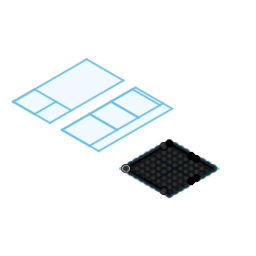
micromouse maze one quarter cutout (Autodesk Fusion 360 design; units mm, degrees)
Autodesk Fusion 360 part; units mm, degrees
sketch "Sketch1" plane through (0, 0, 0) normal (0, 0, 1) x (1, 0, 0)
  line L0 (0, 0) -> (1440, 0)
  line L1 (1440, 0) -> (1440, 1440)
  line L2 (1440, 1440) -> (0, 1440)
  line L3 (0, 1440) -> (0, 0)
  line L4 (720, 1620) -> (720, -180)
  line L5 (0, 0) -> (180, 0)
  line L6 (180, 0) -> (180, 180)
  line L7 (180, 180) -> (0, 180)
  line L8 (0, 180) -> (0, 0)
  line L9 (0, 0) -> (0, -100)
  line L10 (0, -100) -> (-100, -100)
  line L11 (1440, 1440) -> (1540, 1440)
  line L12 (1540, 1440) -> (1540, 1540)
  dimension "d1" = 1440
  dimension "d2" = 1440
  dimension "d7" = 180
  dimension "d8" = 180
  dimension "d9" = 100
  dimension "d10" = 100
  dimension "d11" = 100
  dimension "d12" = 100
  constraint horizontal L0
  constraint vertical L1
  constraint horizontal L2
  constraint vertical L3
  constraint coincident L0.start L3.end
  constraint horizontal L5
  constraint vertical L6
  constraint horizontal L7
  constraint vertical L8
  constraint perpendicular L5 L9
  constraint perpendicular L9 L10
  constraint perpendicular L1 L11
  constraint perpendicular L11 L12
  measures "d1" distance of L0.start L0.end
  measures "d2" distance of L0.start L2.end
  measures "d7" distance of L0.start L5.end
  measures "d8" distance of L0.start L7.end
  measures "d9" distance of L0.start L9.end
  measures "d10" distance of L9.end L10.end
  measures "d11" distance of L1.end L11.end
  measures "d12" distance of L11.end L12.end
extrude "Extrude1" add sketch "Sketch1" along normal blind 12.7
sketch "Sketch2" plane through (0, 0, 12.7) normal (0, 0, 1) x (-1, 0, 0)
  line L0 (0, -1440) -> (0, 0)
  line L1 (0, 0) -> (-1440, 0)
  line L2 (-1440, 0) -> (-1440, -1440)
  line L3 (-1440, -1440) -> (0, -1440)
  line L4 (0, 0) -> (-180, 0)
  line L5 (-180, 0) -> (-360, 0)
  line L6 (-360, 0) -> (-540, 0)
  line L7 (-540, 0) -> (-720, 0)
  line L8 (-720, 0) -> (-720, -1440)
  line L9 (-180, 0) -> (-180, -1440)
  line L10 (-360, 0) -> (-360, -1440)
  line L11 (-540, 0) -> (-540, -1440)
  dimension "d15" = 180
  dimension "d16" = 180
  dimension "d17" = 180
  dimension "d18" = 180
  constraint coincident L0.end L1.start
  constraint perpendicular L0 L4
  constraint perpendicular L0 L5
  constraint parallel L1 L6
  constraint parallel L1 L7
  constraint midpoint L3 L8.end
  constraint coincident L3 L9.end
  constraint perpendicular L3 L9
  constraint coincident L3 L10.end
  constraint perpendicular L3 L10
  constraint coincident L3 L11.end
  constraint perpendicular L3 L11
  measures "d15" distance of L0.end L4.end
  measures "d16" distance of L4.end L5.end
  measures "d17" distance of L5.end L6.end
  measures "d18" distance of L6.end L7.end
sketch "Sketch3" plane through (0, 0, 12.7) normal (0, 0, 1) x (-1, 0, 0)
sketch "Sketch4" plane through (0, 0, 12.7) normal (0, 0, 1) x (-1, 0, 0)
  line L0 (0, 0) -> (-1440, 0)
  line L1 (-1440, 0) -> (-1440, -1440)
  line L2 (-1440, -1440) -> (0, -1440)
  line L3 (0, -1440) -> (0, 0)
  line L4 (-720, 0) -> (-810, 0)
  line L5 (-810, 0) -> (-900, 0)
  line L6 (-900, 0) -> (-1080, 0)
  line L7 (-1080, 0) -> (-1260, 0)
  line L8 (0, 0) -> (0, -180)
  line L9 (0, -180) -> (0, -360)
  line L10 (0, -360) -> (0, -540)
  line L11 (0, -540) -> (0, -720)
  line L12 (0, -720) -> (0, -900)
  line L13 (0, -900) -> (0, -1080)
  line L14 (0, -1080) -> (0, -1260)
  line L15 (-1080, 0) -> (-1260, 0)
  line L16 (0, -180) -> (0, -360)
  line L17 (-720, 0) -> (-810, 0)
  line L18 (0, -1440) -> (0, 0)
  line L19 (0, -1080) -> (0, -1260)
  line L20 (-810, 0) -> (-900, 0)
  line L21 (0, -900) -> (0, -1080)
  line L22 (0, -540) -> (0, -720)
  line L23 (-900, 0) -> (-1080, 0)
  line L24 (0, 0) -> (-1440, 0)
  line L25 (0, 0) -> (0, -180)
  line L26 (-1440, -1440) -> (0, -1440)
  line L27 (0, -720) -> (0, -900)
  line L28 (-1440, 0) -> (-1440, -1440)
  line L29 (0, -360) -> (0, -540)
  line L30 (-1080, 0) -> (-1260, 0)
  line L31 (0, -180) -> (0, -360)
  line L32 (-720, 0) -> (-810, 0)
  line L33 (0, -1440) -> (0, 0)
  line L34 (0, -1080) -> (0, -1260)
  line L35 (-810, 0) -> (-900, 0)
  line L36 (0, -900) -> (0, -1080)
  line L37 (0, -540) -> (0, -720)
  line L38 (-900, 0) -> (-1080, 0)
  line L39 (0, 0) -> (-1440, 0)
  line L40 (0, 0) -> (0, -180)
  line L41 (-1440, -1440) -> (0, -1440)
  line L42 (0, -720) -> (0, -900)
  line L43 (-1440, 0) -> (-1440, -1440)
  line L44 (0, -360) -> (0, -540)
  line L45 (0, -1440) -> (-180, -1440)
  line L46 (-180, -1440) -> (-360, -1440)
  line L47 (-360, -1440) -> (-540, -1440)
  line L48 (-540, -1440) -> (-720, -1440)
  line L49 (90, -1530) -> (-1530, -1530)
  line L50 (-1530, -1530) -> (-1530, 90)
  line L51 (-1530, 90) -> (90, 90)
  line L52 (90, 90) -> (90, -1530)
  line L53 (-720, -1440) -> (-900, -1440)
  line L54 (-1440, -720) -> (-1440, -900)
  line L55 (0, -720) -> (0, -810)
  line L56 (90, 90) -> (-824.4, 90)
  line L57 (-824.4, 90) -> (-824.4, -1530)
  line L58 (-824.4, 90) -> (-1510.2, 90)
  line L59 (90, 90) -> (90, -824.4)
  line L60 (90, -824.4) -> (-1530, -824.4)
  line L61 (2170.8056, -49.2636) -> (951.6056, -49.2636)
  line L62 (951.6056, -49.2636) -> (951.6056, -2487.6636)
  line L63 (951.6056, -2487.6636) -> (2170.8056, -2487.6636)
  line L64 (2170.8056, -2487.6636) -> (2170.8056, -49.2636)
  line L65 (2170.8056, -49.2636) -> (1256.4056, -49.2636)
  line L66 (1256.4056, -49.2636) -> (1256.4056, -963.6636)
  line L67 (1256.4056, -963.6636) -> (2170.8056, -963.6636)
  line L68 (2170.8056, -963.6636) -> (2170.8056, -49.2636)
  line L69 (2170.8056, -963.6636) -> (1256.4056, -963.6636)
  line L70 (1256.4056, -963.6636) -> (1256.4056, -1674.8636)
  line L71 (1256.4056, -1674.8636) -> (2170.8056, -1674.8636)
  line L72 (2170.8056, -1674.8636) -> (2170.8056, -963.6636)
  line L73 (2170.8056, -1674.8636) -> (1256.4056, -1674.8636)
  line L74 (1256.4056, -1674.8636) -> (1256.4056, -2386.0636)
  line L75 (1256.4056, -2386.0636) -> (2170.8056, -2386.0636)
  line L76 (2170.8056, -2386.0636) -> (2170.8056, -1674.8636)
  line L77 (3790.0355, -49.382) -> (2570.8355, -49.382)
  line L78 (2570.8355, -49.382) -> (2570.8355, -2487.782)
  line L79 (2570.8355, -2487.782) -> (3790.0355, -2487.782)
  line L80 (3790.0355, -2487.782) -> (3790.0355, -49.382)
  line L81 (3790.0355, -49.382) -> (3078.8355, -49.382)
  line L82 (3078.8355, -49.382) -> (3078.8355, -760.582)
  line L83 (3078.8355, -760.582) -> (3790.0355, -760.582)
  line L84 (3790.0355, -760.582) -> (3790.0355, -49.382)
  line L85 (1256.4056, -2386.0636) -> (1256.4056, -2487.6636)
  line L86 (3078.8355, -760.582) -> (2570.8355, -760.582)
  point P0 (0, -1440)
  point P1 (-180, -1440)
  point P2 (-360, -1440)
  point P3 (0, -1260)
  point P4 (0, -1080)
  point P5 (0, -900)
  point P6 (0, -720)
  point P7 (0, -540)
  point P8 (0, -360)
  point P9 (0, -180)
  point P10 (-180, -1260)
  point P11 (-180, -1080)
  point P12 (-180, -900)
  point P13 (-180, -720)
  point P14 (-180, -540)
  point P15 (-180, -360)
  point P16 (-180, -180)
  point P17 (-180, 0)
  point P18 (-360, -1260)
  point P19 (-360, -1080)
  point P20 (-360, -900)
  point P21 (-360, -720)
  point P22 (-360, -540)
  point P23 (-360, -360)
  point P24 (-360, -180)
  point P25 (-360, 0)
  point P26 (-540, -1440)
  point P27 (-540, -1260)
  point P28 (-540, -1080)
  point P29 (-540, -900)
  point P30 (-540, -720)
  point P31 (-540, -540)
  point P32 (-540, -360)
  point P33 (-540, -180)
  point P34 (-540, 0)
  point P35 (-720, -1440)
  point P36 (-720, -1260)
  point P37 (-720, -1080)
  point P38 (-720, -900)
  point P39 (-720, -720)
  point P40 (-720, -540)
  point P41 (-720, -360)
  point P42 (-720, -180)
  point P43 (-720, 0)
  point P44 (-900, -1440)
  point P45 (-900, -1260)
  point P46 (-900, -1080)
  point P47 (-900, -900)
  point P48 (-900, -720)
  point P49 (-900, -540)
  point P50 (-900, -360)
  point P51 (-900, -180)
  point P52 (-900, 0)
  point P53 (-1080, -1440)
  point P54 (-1080, -1260)
  point P55 (-1080, -1080)
  point P56 (-1080, -900)
  point P57 (-1080, -720)
  point P58 (-1080, -540)
  point P59 (-1080, -360)
  point P60 (-1080, -180)
  point P61 (-1080, 0)
  point P62 (-1260, -1440)
  point P63 (-1260, -1260)
  point P64 (-1260, -1080)
  point P65 (-1260, -900)
  point P66 (-1260, -720)
  point P67 (-1260, -540)
  point P68 (-1260, -360)
  point P69 (-1260, -180)
  point P70 (-1260, 0)
  point P71 (-1440, -1440)
  point P72 (-1440, -1260)
  point P73 (-1440, -1080)
  point P74 (-1440, -900)
  point P75 (-1440, -720)
  point P76 (-1440, -540)
  point P77 (-1440, -360)
  point P78 (-1440, -180)
  point P79 (-1440, 0)
  dimension "d62" = 1440
  dimension "d63" = 1440
  dimension "d86" = 914.4
  dimension "d90" = 914.4
  dimension "d92" = 1219.2
  dimension "d93" = 2438.4
  dimension "d94" = 914.4
  dimension "d95" = 914.4
  dimension "d96" = 914.4
  dimension "d97" = 711.2
  dimension "d98" = 914.4
  dimension "d99" = 711.2
  dimension "d100" = 1219.2
  dimension "d101" = 2438.4
  dimension "d102" = 711.2
  dimension "d103" = 711.2
  dimension "d105" = 180
  dimension "d106" = 180
  dimension "d107" = 1440
  dimension "d108" = 705.6
  dimension "d109" = 705.6
  constraint coincident L0.start L3.end
  constraint horizontal L0
  constraint vertical L1
  constraint horizontal L2
  constraint vertical L3
  constraint midpoint L0 P43
  constraint coincident L0 L4.end
  constraint perpendicular L0 L8
  constraint horizontal L24
  constraint vertical L28
  constraint horizontal L26
  constraint vertical L18
  constraint midpoint P43 L24
  constraint coincident L4.end L24
  constraint perpendicular L24 L25
  constraint horizontal L39
  constraint vertical L43
  constraint horizontal L41
  constraint vertical L33
  constraint midpoint L4.start L39
  constraint coincident L4.end L39
  constraint perpendicular L39 L40
  constraint perpendicular L33 L45
  constraint parallel L26 L46
  constraint parallel L41 L47
  constraint coincident P0 L2.end
  constraint horizontal L49
  constraint vertical L50
  constraint horizontal L51
  constraint vertical L52
  constraint coincident P35 L48.end
  constraint coincident P44 L53.end
  constraint coincident P75 L54.start
  constraint coincident P74 L54.end
  constraint perpendicular L32 L54
  constraint midpoint L27 L55.end
  constraint parallel L27 L55
  constraint coincident L51 L56.end
  constraint coincident L49 L57.end
  constraint perpendicular L49 L57
  constraint coincident L51 L58.end
  constraint perpendicular L51 L59
  constraint coincident L50 L60.end
  constraint perpendicular L50 L60
  constraint horizontal L61
  constraint vertical L62
  constraint horizontal L63
  constraint vertical L64
  constraint horizontal L65
  constraint vertical L66
  constraint horizontal L67
  constraint vertical L68
  constraint horizontal L69
  constraint vertical L70
  constraint horizontal L71
  constraint vertical L72
  constraint horizontal L73
  constraint vertical L74
  constraint horizontal L75
  constraint vertical L76
  constraint horizontal L77
  constraint vertical L78
  constraint horizontal L79
  constraint vertical L80
  constraint horizontal L81
  constraint vertical L82
  constraint horizontal L83
  constraint vertical L84
  constraint coincident L63 L85.end
  constraint perpendicular L63 L85
  constraint coincident L78 L86.end
  constraint perpendicular L78 L86
  measures "d86" distance of L51.end L56.end
  measures "d90" distance of L51 L60
  measures "d92" distance of L61.start L61.end
  measures "d93" distance of L61.start L63.end
  measures "d94" distance of L61.start L65.end
  measures "d95" distance of L61.start L67.end
  measures "d96" distance of L67.end L66.end
  measures "d97" distance of L67.end L71.end
  measures "d98" distance of L71.end L70.end
  measures "d99" distance of L71.end L75.end
  measures "d100" distance of L77.start L77.end
  measures "d101" distance of L77.start L79.end
  measures "d102" distance of L77.start L81.end
  measures "d103" distance of L77.start L83.end
  measures "d105" distance of P70 P79
  measures "d106" distance of P78 P79
  measures "d107" distance of P79 P71
  measures "d108" distance of L50.end L56.end
  measures "d109" distance of L49.start L59.end
hidden bodies 1
